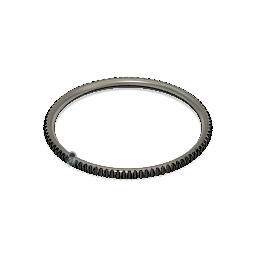
SkjotariV3_PLA v8 (Autodesk Fusion 360 design; units mm, degrees)
Autodesk Fusion 360 part; units mm, degrees
sketch "Sketch1" plane through (0, 0, 0) normal (0, 1, 0) x (1, 0, 0)
  circle A0 centre (0, 0) radius 60
  dimension "d1" = 120
  constraint coincident A0.centre origin
  measures "d1" diameter of A0
extrude "Extrude1" add sketch "Sketch1" along normal blind 12 makes body 1
sketch "Sketch2" plane through (0, 0, 0) normal (0, 0, 1) x (1, 0, 0)
  line L0 (-60, 6) -> (-57.6, 6)
  arc A0 (-60.6, 3) -> (-60.6, 9) centre (-57.6, 6) ccw
  arc A1 (-60.6, 9) -> (-60.6, 3) centre (-57.6, 6) ccw
  constraint horizontal L0
  constraint coincident L0.end A0.centre
revolve "Revolve1" cut sketch "Sketch2" angle 360 about axis through (0, 0, 0) along (0, -1, 0) bodies 1
sketch "Sketch7" plane through (0, 12, 0) normal (0, 1, 0) x (-1, 0, 0)
  circle A0 centre (0, 0) radius 60
  circle A1 centre (0, 0) radius 2.2
  dimension "d45" = 4.4
  constraint coincident A0.centre A1.centre
  measures "d45" diameter of A1
extrude "Extrude9" cut sketch "Sketch7" against normal blind 25 contours A1 bodies 1
sketch "Sketch8" plane through (0, 0, 0) normal (1, 0, 0) x (0, 0, -1)
  ellipse E0 centre (-57, 6) end of major axis (-61, 6) minor radius 4
  line L0 (-53, 6) -> (-61, 6)
  line L1 (-57, 10) -> (-57, 2)
  point P0 (-57, 10)
  constraint horizontal L0
  constraint coincident E0 L0.start
  constraint coincident E0 L0.end
  constraint coincident E0 P0
  constraint coincident E0 L1.end
  constraint coincident P0 L1.start
revolve "Revolve2" add sketch "Sketch8" angle 360 about axis through (0, 12, 0) along (0, 1, 0) separate body makes body 2
sketch "Sketch10" plane through (0, 0, 0) normal (0, 1, 0) x (1, 0, 0)
  line L0 (-67, -4) -> (-57, 0)
  line L1 (-57, 0) -> (-67, 0)
  line L2 (-67, 4) -> (-57, 0)
  line L3 (-67, -4) -> (-67, 4)
  constraint horizontal L1
  constraint symmetric L0.start L1 L2.start
  constraint symmetric L0.end L1 L2.end
extrude "Extrude10" cut sketch "Sketch10" along normal blind 18 bodies 2
fillet "Fillet9" radius 1 1 edges at (-57, 6, 0) on bodies 2
pattern_circular "C-Pattern2" count 90 over 360 about axis through (0, 1.75, 0) along (0, 1, 0) of "Extrude10", "Fillet9"
fillet "Fillet1" [suppressed]
fillet "Fillet2" [suppressed]
fillet "Fillet3" [suppressed]
fillet "Fillet4" [suppressed]
sketch "Sketch4" plane through (0, 12, 0) normal (0, 1, 0) x (-1, 0, 0)
  circle A0 centre (0, 0) radius 59.5
  circle A1 centre (0, 0) radius 1.55
  circle A2 centre (0, 0) radius 59.5
  line L0 (24.3958, 12.8668) -> (35.4895, -15.766)
  line L1 (35.4895, -15.766) -> (31.388, -15.766)
  line L2 (31.388, -15.766) -> (23.9466, 5.0348)
  spline S0 degree 3 poles (23.9466, 5.0348) (23.6636, 5.8395) (23.1191, 7.3882) (22.6622, 8.9649) (22.4427, 9.7223) knots 0 0 0 0 0.25586 0.49237 0.49237 0.49237 0.49237
  spline S1 degree 3 poles (22.4427, 9.7223) (22.2114, 8.9384) (21.7456, 7.3599) (21.183, 5.8133) (20.8997, 5.0348) knots 0 0 0 0 0.24512 0.493597 0.493597 0.493597 0.493597
  line L3 (20.8997, 5.0348) -> (13.1653, -15.766)
  line L4 (13.1653, -15.766) -> (9.2981, -15.766)
  line L5 (9.2981, -15.766) -> (20.5091, 12.8668)
  line L6 (20.5091, 12.8668) -> (24.3958, 12.8668)
  spline S2 degree 3 poles (-18.665, -6.2627) (-18.7707, -6.2513) (-18.959, -6.2311) (-19.1483, -6.2259) (-19.2314, -6.2236) knots 0 0 0 0 0.031873 0.056795 0.056795 0.056795 0.056795
  spline S3 degree 5 poles (-59.1647, -9.9772) (-58.5704, -9.8764) (-57.4132, -9.6642) (-55.7708, -9.3139) (-53.7687, -8.7825) (-51.5831, -8.0102) (-49.7184, -7.1298) (-48.1765, -6.1434) (-46.9546, -5.0564) (-46.0423, -3.8794) (-45.4184, -2.6292) (-45.0583, -1.3277) (-44.9414, 0.0002) (-45.0584, 1.3281) (-45.4187, 2.6295) (-46.0426, 3.8796) (-46.9549, 5.0567) (-48.1767, 6.1438) (-49.7184, 7.1307) (-51.5829, 8.0118) (-53.7683, 8.7851) (-55.7701, 9.3174) (-57.4124, 9.6686) (-58.5696, 9.8815) (-59.1637, 9.9826) knots 0 0 0 0 0 0 0.05 0.1 0.15 0.2 0.25 0.3 0.35 0.4 0.45 0.5 0.55 0.6 0.65 0.7 0.75 0.8 0.85 0.9 0.95 1 1 1 1 1 1
  circle A3 centre (0, 0) radius 60
  line L7 (-59.1647, -9.9772) -> (-59.3128, -10.0023)
  line L8 (-59.1637, 9.9826) -> (-59.3461, 10.0136)
  line L9 (-21.8477, 12.9661) -> (-21.8477, 6.1106)
  line L10 (-21.8477, 6.1106) -> (-9.4258, 6.1106)
  line L11 (-9.4258, 6.1106) -> (-9.4258, 2.888)
  line L12 (-9.4258, 2.888) -> (-22.4922, -15.6667)
  line L13 (-22.4922, -15.6667) -> (-25.3633, -15.6667)
  line L14 (-25.3633, -15.6667) -> (-25.3633, 2.888)
  line L15 (-25.3633, 2.888) -> (-29.2305, 2.888)
  line L16 (-29.2305, 2.888) -> (-29.2305, 6.1106)
  line L17 (-29.2305, 6.1106) -> (-25.3633, 6.1106)
  line L18 (-25.3633, 6.1106) -> (-25.3633, 12.9661)
  line L19 (-25.3633, 12.9661) -> (-21.8477, 12.9661)
  line L20 (-21.8477, 2.888) -> (-21.8477, -10.0222)
  line L21 (-21.8477, -10.0222) -> (-12.8828, 2.888)
  line L22 (-12.8828, 2.888) -> (-21.8477, 2.888)
  point P0 (-47, -5)
  point P1 (-45, 0)
  point P2 (-47, 5)
  dimension "d11" = 3.1
  constraint concentric A0 A1
  constraint coincident S3.start A3
  constraint coincident S3.end A3
  measures "d11" diameter of A1
extrude "Extrude7" [suppressed]
ref_plane "WorkPlane1" through (-0.4152, 6, 0.0022) normal (0, 1, 0) x (-1, 0, 0)
mirror "Mirror2" [suppressed]
extrude "Extrude5" [suppressed]
extrude "Extrude8" [suppressed]
extrude "Extrude3" [suppressed]
extrude "Extrude4" [suppressed]
sketch "Sketch6" plane through (0, 0, 0) normal (0, -1, 0) x (1, 0, 0)
  circle A0 centre (0, 0) radius 1.55
  arc A1 (58.6712, 9.8966) -> (58.6721, -9.8914) centre (0, 0) ccw
  spline S0 degree 3 poles (58.6712, 9.8966) (56.0942, 9.4345) (52.3324, 8.5922) (48.1485, 6.1457) (47.2039, 5.3188) (45.8131, 3.5261) (45.4526, 2.6466) (45.0133, 1.0292) (44.9445, 0.0991) (45.1262, -1.5539) (45.344, -2.4957) (46.3784, -4.3665) (47.0387, -5.1192) (48.9464, -6.7158) (50.3173, -7.4352) (54.0966, -8.9739) (56.7187, -9.5423) (58.6721, -9.8914) knots 0.118723 0.118723 0.118723 0.118723 0.742092 0.742092 1.02193 1.02193 1.311544 1.311544 1.660435 1.660435 1.947559 1.947559 2.204945 2.204945 2.580611 2.580611 3.247512 3.247512 3.247512 3.247512
pattern_circular "C-Pattern1" [suppressed]
fillet "Fillet5" [suppressed]
fillet "Fillet6" [suppressed]
fillet "Fillet7" [suppressed]
fillet "Fillet8" [suppressed]
hidden bodies 1
